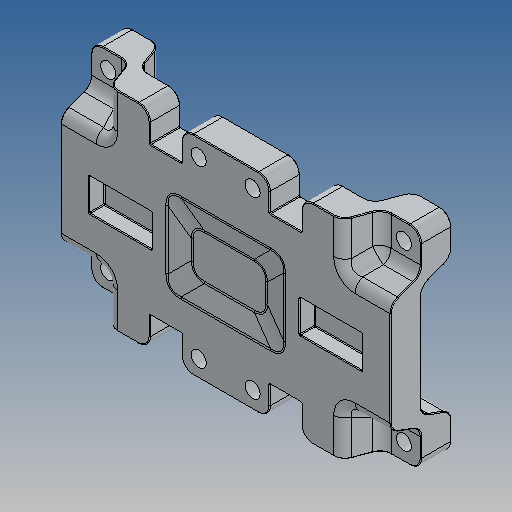
# Autodesk Inventor part: 84428-LtBluishGray
Saved by Autodesk Inventor 2025 (Build 290162010, 162A)
## iProperties
Created: 2024-11-28
Part Number: 84428-LtBluishGray
Material: ABS-Kunststoff
Document SubType Name: Modeling
Designer: hp.muther
Density: 1.06 g/cm^3
Appearance: LtBluishGray
Author: hp.muther
Autodesk Inventor part; units mm, degrees
(part 1 of 2)
ref_plane "YZ Plane" through (0, 0, 0) normal (1, 0, 0) x (0, 1, 0)
ref_plane "XZ Plane" through (0, 0, 0) normal (0, 1, 0) x (-1, 0, 0)
ref_plane "XY Plane" through (0, 0, 0) normal (0, 0, 1) x (1, 0, 0)
sketch "Skizze1" plane through (0, 0, 0) normal (0, 1, 0) x (-1, 0, 0)
  line L0 (0, 0) -> (0, 27.5)
  line L1 (0, 27.5) -> (43.5, 27.5)
  line L2 (43.5, 27.5) -> (43.5, 0)
  line L3 (43.5, 0) -> (0, 0)
  dimension "d0" = 27.5
  dimension "d1" = 43.5
  constraints: 8 end point, 3 perpendicular, 1 vertical
  measures "d0" distance of L0.start L0.end
  measures "d1" distance of L2.end L0.start
extrude "Extrusion1" add sketch "Skizze1" along normal blind 8
sketch "Skizze2" plane through (0, 8, 0) normal (0, 1, 0) x (1, 0, 0)
  line L0 (-43.5, 0) -> (-43.5, -27.5) projected
  line L1 (-43.5, -27.5) -> (0, -27.5) projected
  line L2 (-43.5, -27.5) -> (-30.5882, -27.5)
  line L3 (-30.5882, -27.5) -> (-30.5882, -14.5882)
  line L4 (-30.5882, -14.5882) -> (-43.5, -14.5882)
  line L5 (-43.5, -14.5882) -> (-43.5, -27.5)
  line L6 (-30.5882, -19.5) -> (-33.5, -27.5) construction
  point P0 (-43.5, -14.5882)
  dimension "d4" = 12.9118
  dimension "d10" = 20
  dimension "d11" = 8
  dimension "d12" = 10
  constraints: 10 end point, 2 parallel, 2 perpendicular, 2 point on line, 1 horizontal
  measures "d4" distance of L3.end L4.end
  measures "d10" angle of L3 L6
  measures "d11" vertical distance of L6.start L6.end
  measures "d12" distance from line of L6.end L0
extrude "Extrusion2" add sketch "Skizze2" along normal blind 8
draft "Flächenverjüngung1" angle 20 pull direction (0, 1, 0) faces at (-34.8922, 10.6667, 14.5882) (-30.5882, 10.6667, 23.1961) fixed edges at (-37.0441, 8, 14.5882) (-30.5882, 8, 21.0441)
sketch "Skizze3" plane through (0, 8, 0) normal (0, 1, 0) x (1, 0, 0)
  line L0 (-43.5, -27.5) -> (-33.5, -27.5)
  line L1 (-33.5, -27.5) -> (-33.5, -17.5)
  line L2 (-33.5, -17.5) -> (-43.5, -17.5)
  line L3 (-43.5, -17.5) -> (-43.5, -27.5)
  dimension "d13" = 10
  constraints: 8 end point, 2 parallel, 2 perpendicular, 1 horizontal
  measures "d13" distance of L1.end L2.end
extrude "Extrusion3" cut sketch "Skizze3" against normal blind 8 draft 20
sketch "Skizze4" plane through (0, 0, 0) normal (0, -1, 0) x (1, 0, 0)
  line L0 (0, 0) -> (-43.5, 0) projected
  line L1 (0, 27.5) -> (0, 0) projected
  line L2 (-30.5882, 27.5) -> (0, 27.5) projected
  line L3 (-11.6, 27.5) -> (-20, 27.5)
  line L4 (-20, 27.5) -> (-20, 19.5)
  line L5 (-20, 19.5) -> (-11.6, 19.5)
  line L6 (-11.6, 19.5) -> (-11.6, 27.5)
  dimension "d16" = 19.5
  dimension "d17" = 8.4
  dimension "d18" = 20
  constraints: 8 end point, 2 parallel, 1 horizontal, 1 perpendicular, 1 point on line
  measures "d16" distance between parallel lines of L5 L0
  measures "d17" distance between parallel lines of L6 L4
  measures "d18" distance between parallel lines of L4 L1
extrude "Extrusion4" cut sketch "Skizze4" against normal through all
sketch "Skizze5" plane through (0, 0, 0) normal (0, -1, 0) x (1, 0, 0)
  line L0 (0, 0) -> (-43.5, 0) projected
  line L1 (0, 27.5) -> (0, 0) projected
  line L2 (-36, 0) -> (-19.5, 0)
  line L3 (-19.5, 0) -> (-19.5, 4.25)
  line L4 (-19.5, 4.25) -> (-36, 4.25)
  line L5 (-36, 4.25) -> (-36, 0)
  circle A0 centre (-7.1, 23) radius 2
  line L6 (-11.6, 27.5) -> (0, 27.5) projected
  line L7 (-11.6, 27.5) -> (-11.6, 19.5) projected
  dimension "d21" = 16.5
  dimension "d22" = 4.25
  dimension "d23" = 36
  dimension "d26" = 4
  dimension "d46" = 4.5
  dimension "d47" = 4.5
  constraints: 8 end point, 2 parallel, 1 centre point, 1 horizontal, 1 perpendicular, 1 point on line
  measures "d21" distance of L3.end L4.end
  measures "d22" distance between parallel lines of L0 L4
  measures "d23" distance between parallel lines of L5 L1
  measures "d26" diameter of A0
  measures "d46" distance from line of A0.centre L6
  measures "d47" distance from line of A0.centre L7
extrude "Extrusion5" cut sketch "Skizze5" against normal blind 4
sketch "Skizze6" plane through (0, 0, 0) normal (0, -1, 0) x (1, 0, 0)
  line L0 (0, 0) -> (-19.5, 0) projected
  line L1 (0, 27.5) -> (0, 0) projected
  line L2 (0, 0) -> (-9.8287, 0)
  line L3 (-9.8287, 0) -> (-9.8287, 5.8287)
  line L4 (-9.8287, 5.8287) -> (0, 5.8287)
  line L5 (0, 5.8287) -> (0, 0)
  line L6 (0, 0) -> (-15.5, 0)
  line L7 (-15.5, 0) -> (-15.5, 11.5)
  line L8 (-15.5, 11.5) -> (0, 11.5)
  line L9 (0, 11.5) -> (0, 0)
  line L10 (-15.5, 0) -> (-9.8287, 1)
  point P0 (0, 5.8287)
  point P1 (-9.8287, 0)
  dimension "d29" = 9.8287
  dimension "d30" = 5.8287
  dimension "d34" = 11.5
  dimension "d35" = 15.5
  dimension "d36" = 10
  dimension "d37" = 1
  dimension "d38" = 7.5475
  dimension "d39" = 5.6713
  constraints: 18 end point, 4 parallel, 2 horizontal, 2 perpendicular, 1 point on line
  measures "d29" distance of L3.end L4.end
  measures "d30" distance of L2.end L3.end
  measures "d34" distance between parallel lines of L0 L8
  measures "d35" distance between parallel lines of L9 L7
  measures "d36" angle of L6 L10
  measures "d37" distance from line of L0 L10.end
  measures "d39" distance between parallel lines of L8 L4
extrude "Extrusion6" cut sketch "Skizze6" against normal blind 1 contours L0 L3 L4 L1
draft "Flächenverjüngung2" angle 80 pull direction (0, -1, 0) faces at (-9.8287, 0.3333, 3.8858) (-3.2762, 0.6667, 5.8287) fixed edges at (-9.8287, 1, 2.9144) (-4.9144, 1, 5.8287)
fillet "Rundung1" radius 20 1 edges at (-12.6644, 0.5, 8.6644)
mirror "Spiegeln1" about plane through (-7.1, 4, 23) normal (0, -1, 0) of "Extrusion6", "Flächenverjüngung2", "Rundung1"
sketch "Skizze7" plane through (0, 8, 0) normal (0, -1, 0) x (1, 0, 0)
  line L0 (-43.5, 27.5) -> (-33.5, 27.5) projected
  line L1 (-43.5, 17.5) -> (-43.5, 27.5) projected
  circle A0 centre (-39, 23) radius 2
  point P0 (0, 0)
  dimension "d41" = 4
  dimension "d42" = 4.5
  dimension "d43" = 4.5
  constraints: 1 centre point
  measures "d41" diameter of A0
  measures "d42" distance from line of A0.centre L1
  measures "d43" distance from line of A0.centre L0
extrude "Extrusion7" cut sketch "Skizze7" against normal blind 4
fillet "Rundung2" radius 3 25 edges at (-30.5882, 8, 21.0441) (-37.0441, 8, 14.5882) (-32.0441, 12, 16.0441) (-38.5, 16, 17.5) (-33.5, 16, 22.5) (-38.5, 8, 17.5) (-33.5, 8, 22.5) (-32.0441, 4, 16.0441) (-30.5882, 0, 21.0441) (-37.0441, 0, 14.5882) (-43.5, 12, 27.5) (-20, 4, 27.5) (-11.6, 4, 27.5) (-14.6285, 8, 10.6285) (-15.5, 8, 4.0135) (-6.0135, 8, 11.5) (-3.1779, 7, 5.8287) (-9.8287, 7, 1.1779) (-8.9572, 7, 4.9572) (-15.5, 0, 4.0135) (-6.0135, 0, 11.5) (-14.6285, 0, 10.6285) (-9.8287, 1, 1.1779) (-3.1779, 1, 5.8287) (-8.9572, 1, 4.9572)
fillet "Rundung2" radius 0.2 4 edges at (-20, 4, 19.5) (-11.6, 4, 19.5) (-19.5, 2, 4.25) (-36, 2, 4.25)
fillet "Rundung3" radius 0.2 48 edges at (-20.8787, 8, 26.6213) (-20, 8, 22.1) (-19.9414, 8, 19.5586) (-15.8, 8, 19.5) (-11.6586, 8, 19.5586) (-11.6, 8, 22.1) (-10.7213, 8, 26.6213) (-4.3, 8, 27.5) (-30.2083, 8.5425, 27.5) (-32.0441, 12, 27.5) (-33.8799, 15.4575, 27.5) (-38.0503, 16, 27.5) (-42.6213, 16, 26.6213) (-43.5, 16, 22.0503) (-43.5, 15.4575, 17.8799) (-43.5, 12, 16.0441) (-43.5, 8.5425, 14.2083) (-43.5, 8, 6.2438) (-25.7438, 8, 27.5) (-20.8787, 0, 26.6213) (-20, 0, 22.1) (-19.9414, 0, 19.5586) (-15.8, 0, 19.5) (-11.6586, 0, 19.5586) (-11.6, 0, 22.1) (-10.7213, 0, 26.6213) (-4.3, 0, 27.5) (-30.2083, 0.5425, 27.5) (-32.0441, 4, 27.5) (-33.8799, 7.4575, 27.5) (-38.0503, 8, 27.5) (-42.6213, 8, 26.6213) (-43.5, 8, 22.0503) (-43.5, 7.4575, 17.8799) (-43.5, 4, 16.0441) (-43.5, 0.5425, 14.2083) (-43.5, 0, 6.2438) (-25.7438, 0, 27.5) (-19.5586, 0, 4.1914) (-19.5, 0, 2.025) (-35.9414, 0, 4.1914) (-36, 0, 2.025) (-27.75, 0, 4.25) (-19.5586, 4, 4.1914) (-19.5, 4, 2.025) (-35.9414, 4, 4.1914) (-36, 4, 2.025) (-27.75, 4, 4.25)
mirror "Spiegeln2" about plane through (0, 0, 0) normal (0, 0, -1)
mirror "Spiegeln3" about plane through (0, 0, 27.5) normal (1, 0, 0)
sketch "Skizze8" plane through (0, 8, 0) normal (0, 1, 0) x (1, 0, 0)
  line L0 (-32, -5) -> (-42, -5)
  line L1 (-42, -5) -> (-42, 5)
  line L2 (-42, 5) -> (-32, 5)
  line L3 (-32, 5) -> (-32, -5)
  line L4 (-41.9167, -4.9167) -> (-41.9167, 4.9167)
  line L5 (-41.9167, 4.9167) -> (-32.0833, 4.9167)
  line L6 (-32.0833, 4.9167) -> (-32.0833, -4.9167)
  line L7 (-32.0833, -4.9167) -> (-41.9167, -4.9167)
  spline S0 degree 3 poles (-35.473, -0.7347) (-35.3624, -0.6395) (-35.2195, -0.4588) (-35.1278, -0.1698) (-35.0916, 0.0842) (-35.1043, 0.3702) (-35.1747, 0.6728) (-35.3516, 1.0506) (-35.5547, 1.2912) (-35.7186, 1.4187) knots 0 0 0 0 0.178983 0.273938 0.368222 0.492079 0.622193 0.746013 1 1 1 1
  line L8 (-35.473, -0.7347) -> (-35.3624, -0.6395) construction
  line L9 (-35.3624, -0.6395) -> (-35.2195, -0.4588) construction
  line L10 (-35.2195, -0.4588) -> (-35.1278, -0.1698) construction
  line L11 (-35.1278, -0.1698) -> (-35.0916, 0.0842) construction
  line L12 (-35.0916, 0.0842) -> (-35.1043, 0.3702) construction
  line L13 (-35.1043, 0.3702) -> (-35.1747, 0.6728) construction
  line L14 (-35.1747, 0.6728) -> (-35.3516, 1.0506) construction
  line L15 (-35.3516, 1.0506) -> (-35.5547, 1.2912) construction
  line L16 (-35.5547, 1.2912) -> (-35.7186, 1.4187) construction
  spline S1 degree 3 poles (-35.3027, 1.3649) (-35.2254, 1.2746) (-35.09, 1.0821) (-34.9632, 0.8118) (-34.8957, 0.5786) (-34.8526, 0.3435) (-34.8424, 0.119) (-34.8636, -0.0901) (-34.8884, -0.224) (-34.9248, -0.3582) (-34.9903, -0.5271) (-35.0674, -0.6551) (-35.1272, -0.7328) (-35.137, -0.7452) knots 0 0 0 0 0.159789 0.316619 0.39902 0.481421 0.638299 0.698008 0.757718 0.817853 0.877988 0.980322 1 1 1 1
  line L17 (-35.3027, 1.3649) -> (-35.2254, 1.2746) construction
  line L18 (-35.2254, 1.2746) -> (-35.09, 1.0821) construction
  line L19 (-35.09, 1.0821) -> (-34.9632, 0.8118) construction
  line L20 (-34.9632, 0.8118) -> (-34.8957, 0.5786) construction
  line L21 (-34.8957, 0.5786) -> (-34.8526, 0.3435) construction
  line L22 (-34.8526, 0.3435) -> (-34.8424, 0.119) construction
  line L23 (-34.8424, 0.119) -> (-34.8636, -0.0901) construction
  line L24 (-34.8636, -0.0901) -> (-34.8884, -0.224) construction
  line L25 (-34.8884, -0.224) -> (-34.9248, -0.3582) construction
  line L26 (-34.9248, -0.3582) -> (-34.9903, -0.5271) construction
  line L27 (-34.9903, -0.5271) -> (-35.0674, -0.6551) construction
  line L28 (-35.0674, -0.6551) -> (-35.1272, -0.7328) construction
  line L29 (-35.1272, -0.7328) -> (-35.137, -0.7452) construction
  spline S2 degree 3 poles (-38.4765, 2.1644) (-38.496, 2.156) (-38.5452, 2.1307) (-38.6253, 2.0736) (-38.7157, 1.9854) (-38.8087, 1.8699) (-38.8816, 1.7254) (-38.9348, 1.5546) (-38.9716, 1.3719) (-38.9833, 1.1731) (-38.9859, 0.9738) (-38.959, 0.783) (-38.9219, 0.6128) (-38.8748, 0.4674) (-38.8227, 0.3417) (-38.748, 0.2091) (-38.682, 0.1256) (-38.6415, 0.0726) knots 0 0 0 0 0.027057 0.070486 0.124946 0.187916 0.258874 0.330051 0.415845 0.496025 0.584026 0.669773 0.741314 0.806204 0.86459 0.914785 1 1 1 1
  line L30 (-38.4765, 2.1644) -> (-38.496, 2.156) construction
  line L31 (-38.496, 2.156) -> (-38.5452, 2.1307) construction
  line L32 (-38.5452, 2.1307) -> (-38.6253, 2.0736) construction
  line L33 (-38.6253, 2.0736) -> (-38.7157, 1.9854) construction
  line L34 (-38.7157, 1.9854) -> (-38.8087, 1.8699) construction
  line L35 (-38.8087, 1.8699) -> (-38.8816, 1.7254) construction
  line L36 (-38.8816, 1.7254) -> (-38.9348, 1.5546) construction
  line L37 (-38.9348, 1.5546) -> (-38.9716, 1.3719) construction
  line L38 (-38.9716, 1.3719) -> (-38.9833, 1.1731) construction
  line L39 (-38.9833, 1.1731) -> (-38.9859, 0.9738) construction
  line L40 (-38.9859, 0.9738) -> (-38.959, 0.783) construction
  line L41 (-38.959, 0.783) -> (-38.9219, 0.6128) construction
  line L42 (-38.9219, 0.6128) -> (-38.8748, 0.4674) construction
  line L43 (-38.8748, 0.4674) -> (-38.8227, 0.3417) construction
  line L44 (-38.8227, 0.3417) -> (-38.748, 0.2091) construction
  line L45 (-38.748, 0.2091) -> (-38.682, 0.1256) construction
  line L46 (-38.682, 0.1256) -> (-38.6415, 0.0726) construction
  spline S3 degree 3 poles (-38.973, 0.104) (-38.9979, 0.1432) (-39.0496, 0.2355) (-39.0988, 0.3548) (-39.1347, 0.4582) (-39.1607, 0.5455) (-39.1829, 0.6361) (-39.2024, 0.7334) (-39.2194, 0.8381) (-39.2317, 0.9573) (-39.2347, 1.0772) (-39.2319, 1.1851) (-39.227, 1.2895) (-39.2167, 1.4009) (-39.1978, 1.5159) (-39.1663, 1.6523) (-39.1252, 1.7852) (-39.0668, 1.9143) (-39.0137, 2.0064) (-38.9537, 2.0889) (-38.9024, 2.1484) (-38.8687, 2.1839) (-38.8557, 2.1969) knots 0 0 0 0 0.059837 0.132225 0.172452 0.212678 0.257027 0.301377 0.354532 0.407687 0.46224 0.516793 0.566497 0.616202 0.669387 0.722571 0.810819 0.854806 0.898794 0.93783 0.976866 1 1 1 1
  line L47 (-38.973, 0.104) -> (-38.9979, 0.1432) construction
  line L48 (-38.9979, 0.1432) -> (-39.0496, 0.2355) construction
  line L49 (-39.0496, 0.2355) -> (-39.0988, 0.3548) construction
  line L50 (-39.0988, 0.3548) -> (-39.1347, 0.4582) construction
  line L51 (-39.1347, 0.4582) -> (-39.1607, 0.5455) construction
  line L52 (-39.1607, 0.5455) -> (-39.1829, 0.6361) construction
  line L53 (-39.1829, 0.6361) -> (-39.2024, 0.7334) construction
  line L54 (-39.2024, 0.7334) -> (-39.2194, 0.8381) construction
  line L55 (-39.2194, 0.8381) -> (-39.2317, 0.9573) construction
  line L56 (-39.2317, 0.9573) -> (-39.2347, 1.0772) construction
  line L57 (-39.2347, 1.0772) -> (-39.2319, 1.1851) construction
  line L58 (-39.2319, 1.1851) -> (-39.227, 1.2895) construction
  line L59 (-39.227, 1.2895) -> (-39.2167, 1.4009) construction
  line L60 (-39.2167, 1.4009) -> (-39.1978, 1.5159) construction
  line L61 (-39.1978, 1.5159) -> (-39.1663, 1.6523) construction
  line L62 (-39.1663, 1.6523) -> (-39.1252, 1.7852) construction
  line L63 (-39.1252, 1.7852) -> (-39.0668, 1.9143) construction
  line L64 (-39.0668, 1.9143) -> (-39.0137, 2.0064) construction
  line L65 (-39.0137, 2.0064) -> (-38.9537, 2.0889) construction
  line L66 (-38.9537, 2.0889) -> (-38.9024, 2.1484) construction
  line L67 (-38.9024, 2.1484) -> (-38.8687, 2.1839) construction
  line L68 (-38.8687, 2.1839) -> (-38.8557, 2.1969) construction
  spline S4 degree 3 poles (-36.653, 0.7792) (-36.6576, 0.6963) (-36.7122, 0.5242) (-36.8901, 0.5099) (-36.9901, 0.5385) (-37.0893, 0.5769) (-37.1802, 0.6371) (-37.2609, 0.726) (-37.3082, 0.8385) (-37.3294, 0.9568) (-37.3399, 1.0766) (-37.339, 1.2043) (-37.3177, 1.3389) (-37.2557, 1.4577) (-37.1613, 1.5412) (-37.0413, 1.5828) (-36.9075, 1.5817) (-36.7579, 1.5657) (-36.5824, 1.5258) (-36.391, 1.4628) (-36.1893, 1.374) (-35.9783, 1.2471) (-35.7808, 1.0856) (-35.6257, 0.8856) (-35.5009, 0.6796) (-35.43, 0.4656) (-35.4032, 0.2478) (-35.3962, 0.0501) (-35.4357, -0.1532) (-35.5185, -0.3428) (-35.6607, -0.5088) (-35.8941, -0.634) (-36.1782, -0.6714) (-36.4895, -0.6312) (-36.7559, -0.5759) (-37.0415, -0.4903) (-37.2985, -0.3989) (-37.5745, -0.2896) (-37.8049, -0.1786) (-38.0112, -0.0619) (-38.1801, 0.0538) (-38.3524, 0.1963) (-38.4952, 0.3757) (-38.6003, 0.5957) (-38.656, 0.8014) (-38.6787, 1.0207) (-38.672, 1.2395) (-38.6426, 1.471) (-38.5689, 1.6832) (-38.4342, 1.8427) (-38.2496, 1.9328) (-38.0438, 1.9273) (-37.8337, 1.893) (-37.655, 1.7906) (-37.5297, 1.6397) (-37.4854, 1.4696) (-37.4764, 1.317) (-37.5071, 1.1986) (-37.5522, 1.1238) (-37.6077, 1.0813) (-37.6746, 1.0656) (-37.7498, 1.0726) (-37.8285, 1.0877) (-37.8988, 1.1301) (-37.9872, 1.1175) (-38.024, 1.0355) (-38.0262, 0.9522) (-38.0081, 0.8654) (-37.9569, 0.7893) (-37.8896, 0.7032) (-37.7734, 0.6342) (-37.6311, 0.5633) (-37.4707, 0.4893) (-37.2636, 0.4036) (-37.021, 0.3163) (-36.746, 0.2176) (-36.5084, 0.1557) (-36.3238, 0.1341) (-36.193, 0.1683) (-36.1433, 0.28) (-36.1489, 0.4008) (-36.2089, 0.5256) (-36.3468, 0.6608) (-36.4774, 0.7295) (-36.5685, 0.7576) knots 0 0 0 0 0.019628 0.027018 0.033965 0.040941 0.048656 0.056022 0.065138 0.073134 0.080528 0.089672 0.099198 0.108096 0.11648 0.124306 0.133455 0.143566 0.155056 0.170131 0.184678 0.199975 0.220335 0.236354 0.251449 0.269379 0.28185 0.296238 0.309598 0.323802 0.338076 0.353381 0.376853 0.395227 0.417369 0.432365 0.456106 0.473078 0.492988 0.508303 0.521448 0.534776 0.553874 0.56769 0.58436 0.597126 0.612617 0.628953 0.644733 0.657749 0.670618 0.685183 0.698991 0.713855 0.726199 0.737953 0.749129 0.757115 0.762561 0.766674 0.771046 0.776214 0.782044 0.787215 0.792824 0.7976 0.804046 0.809875 0.815303 0.822628 0.832017 0.842463 0.855224 0.868048 0.888264 0.907855 0.927805 0.938062 0.946095 0.95306 0.961017 0.970332 0.980566 1 1 1 1
  line L69 (-36.653, 0.7792) -> (-36.6576, 0.6963) construction
  line L70 (-36.6576, 0.6963) -> (-36.7122, 0.5242) construction
  line L71 (-36.7122, 0.5242) -> (-36.8901, 0.5099) construction
  line L72 (-36.8901, 0.5099) -> (-36.9901, 0.5385) construction
  line L73 (-36.9901, 0.5385) -> (-37.0893, 0.5769) construction
  line L74 (-37.0893, 0.5769) -> (-37.1802, 0.6371) construction
  line L75 (-37.1802, 0.6371) -> (-37.2609, 0.726) construction
  line L76 (-37.2609, 0.726) -> (-37.3082, 0.8385) construction
  line L77 (-37.3082, 0.8385) -> (-37.3294, 0.9568) construction
  line L78 (-37.3294, 0.9568) -> (-37.3399, 1.0766) construction
  line L79 (-37.3399, 1.0766) -> (-37.339, 1.2043) construction
  line L80 (-37.339, 1.2043) -> (-37.3177, 1.3389) construction
  line L81 (-37.3177, 1.3389) -> (-37.2557, 1.4577) construction
  line L82 (-37.2557, 1.4577) -> (-37.1613, 1.5412) construction
  line L83 (-37.1613, 1.5412) -> (-37.0413, 1.5828) construction
  line L84 (-37.0413, 1.5828) -> (-36.9075, 1.5817) construction
  line L85 (-36.9075, 1.5817) -> (-36.7579, 1.5657) construction
  line L86 (-36.7579, 1.5657) -> (-36.5824, 1.5258) construction
  line L87 (-36.5824, 1.5258) -> (-36.391, 1.4628) construction
  line L88 (-36.391, 1.4628) -> (-36.1893, 1.374) construction
  line L89 (-36.1893, 1.374) -> (-35.9783, 1.2471) construction
  line L90 (-35.9783, 1.2471) -> (-35.7808, 1.0856) construction
  line L91 (-35.7808, 1.0856) -> (-35.6257, 0.8856) construction
  line L92 (-35.6257, 0.8856) -> (-35.5009, 0.6796) construction
  line L93 (-35.5009, 0.6796) -> (-35.43, 0.4656) construction
  line L94 (-35.43, 0.4656) -> (-35.4032, 0.2478) construction
  line L95 (-35.4032, 0.2478) -> (-35.3962, 0.0501) construction
  line L96 (-35.3962, 0.0501) -> (-35.4357, -0.1532) construction
  line L97 (-35.4357, -0.1532) -> (-35.5185, -0.3428) construction
  line L98 (-35.5185, -0.3428) -> (-35.6607, -0.5088) construction
  line L99 (-35.6607, -0.5088) -> (-35.8941, -0.634) construction
  line L100 (-35.8941, -0.634) -> (-36.1782, -0.6714) construction
  line L101 (-36.1782, -0.6714) -> (-36.4895, -0.6312) construction
  line L102 (-36.4895, -0.6312) -> (-36.7559, -0.5759) construction
  line L103 (-36.7559, -0.5759) -> (-37.0415, -0.4903) construction
  line L104 (-37.0415, -0.4903) -> (-37.2985, -0.3989) construction
  line L105 (-37.2985, -0.3989) -> (-37.5745, -0.2896) construction
  line L106 (-37.5745, -0.2896) -> (-37.8049, -0.1786) construction
  line L107 (-37.8049, -0.1786) -> (-38.0112, -0.0619) construction
  line L108 (-38.0112, -0.0619) -> (-38.1801, 0.0538) construction
  line L109 (-38.1801, 0.0538) -> (-38.3524, 0.1963) construction
  line L110 (-38.3524, 0.1963) -> (-38.4952, 0.3757) construction
  line L111 (-38.4952, 0.3757) -> (-38.6003, 0.5957) construction
  line L112 (-38.6003, 0.5957) -> (-38.656, 0.8014) construction
  line L113 (-38.656, 0.8014) -> (-38.6787, 1.0207) construction
  line L114 (-38.6787, 1.0207) -> (-38.672, 1.2395) construction
  line L115 (-38.672, 1.2395) -> (-38.6426, 1.471) construction
  line L116 (-38.6426, 1.471) -> (-38.5689, 1.6832) construction
  line L117 (-38.5689, 1.6832) -> (-38.4342, 1.8427) construction
  line L118 (-38.4342, 1.8427) -> (-38.2496, 1.9328) construction
  line L119 (-38.2496, 1.9328) -> (-38.0438, 1.9273) construction
  line L120 (-38.0438, 1.9273) -> (-37.8337, 1.893) construction
  line L121 (-37.8337, 1.893) -> (-37.655, 1.7906) construction
  line L122 (-37.655, 1.7906) -> (-37.5297, 1.6397) construction
  line L123 (-37.5297, 1.6397) -> (-37.4854, 1.4696) construction
  line L124 (-37.4854, 1.4696) -> (-37.4764, 1.317) construction
  line L125 (-37.4764, 1.317) -> (-37.5071, 1.1986) construction
  line L126 (-37.5071, 1.1986) -> (-37.5522, 1.1238) construction
  line L127 (-37.5522, 1.1238) -> (-37.6077, 1.0813) construction
  line L128 (-37.6077, 1.0813) -> (-37.6746, 1.0656) construction
  line L129 (-37.6746, 1.0656) -> (-37.7498, 1.0726) construction
  line L130 (-37.7498, 1.0726) -> (-37.8285, 1.0877) construction
  line L131 (-37.8285, 1.0877) -> (-37.8988, 1.1301) construction
  line L132 (-37.8988, 1.1301) -> (-37.9872, 1.1175) construction
  line L133 (-37.9872, 1.1175) -> (-38.024, 1.0355) construction
  line L134 (-38.024, 1.0355) -> (-38.0262, 0.9522) construction
  line L135 (-38.0262, 0.9522) -> (-38.0081, 0.8654) construction
  line L136 (-38.0081, 0.8654) -> (-37.9569, 0.7893) construction
  line L137 (-37.9569, 0.7893) -> (-37.8896, 0.7032) construction
  line L138 (-37.8896, 0.7032) -> (-37.7734, 0.6342) construction
  line L139 (-37.7734, 0.6342) -> (-37.6311, 0.5633) construction
  line L140 (-37.6311, 0.5633) -> (-37.4707, 0.4893) construction
  line L141 (-37.4707, 0.4893) -> (-37.2636, 0.4036) construction
  line L142 (-37.2636, 0.4036) -> (-37.021, 0.3163) construction
  line L143 (-37.021, 0.3163) -> (-36.746, 0.2176) construction
  line L144 (-36.746, 0.2176) -> (-36.5084, 0.1557) construction
  line L145 (-36.5084, 0.1557) -> (-36.3238, 0.1341) construction
  line L146 (-36.3238, 0.1341) -> (-36.193, 0.1683) construction
  line L147 (-36.193, 0.1683) -> (-36.1433, 0.28) construction
  line L148 (-36.1433, 0.28) -> (-36.1489, 0.4008) construction
  line L149 (-36.1489, 0.4008) -> (-36.2089, 0.5256) construction
  line L150 (-36.2089, 0.5256) -> (-36.3468, 0.6608) construction
  line L151 (-36.3468, 0.6608) -> (-36.4774, 0.7295) construction
  line L152 (-36.4774, 0.7295) -> (-36.5685, 0.7576) construction
  spline S5 degree 3 poles (-36.5685, 0.7576) (-36.4774, 0.7295) (-36.3468, 0.6608) (-36.2089, 0.5256) (-36.1489, 0.4008) (-36.1433, 0.28) (-36.193, 0.1683) (-36.3238, 0.1341) (-36.5084, 0.1557) (-36.746, 0.2176) (-37.021, 0.3163) (-37.2636, 0.4036) (-37.4707, 0.4893) (-37.6311, 0.5633) (-37.7734, 0.6342) (-37.8896, 0.7032) (-37.9569, 0.7893) (-38.0081, 0.8654) (-38.0262, 0.9522) (-38.024, 1.0355) (-37.9872, 1.1175) (-37.8988, 1.1301) (-37.8285, 1.0877) (-37.7498, 1.0726) (-37.6746, 1.0656) (-37.6077, 1.0813) (-37.5522, 1.1238) (-37.5071, 1.1986) (-37.4764, 1.317) (-37.4854, 1.4696) (-37.5297, 1.6397) (-37.655, 1.7906) (-37.8337, 1.893) (-38.0438, 1.9273) (-38.2496, 1.9328) (-38.4342, 1.8427) (-38.5689, 1.6832) (-38.6426, 1.471) (-38.672, 1.2395) (-38.6787, 1.0207) (-38.656, 0.8014) (-38.6003, 0.5957) (-38.4952, 0.3757) (-38.3524, 0.1963) (-38.1801, 0.0538) (-38.0112, -0.0619) (-37.8049, -0.1786) (-37.5745, -0.2896) (-37.2985, -0.3989) (-37.0415, -0.4903) (-36.7559, -0.5759) (-36.4895, -0.6312) (-36.1782, -0.6714) (-35.8941, -0.634) (-35.6607, -0.5088) (-35.5185, -0.3428) (-35.4357, -0.1532) (-35.3962, 0.0501) (-35.4032, 0.2478) (-35.43, 0.4656) (-35.5009, 0.6796) (-35.6257, 0.8856) (-35.7808, 1.0856) (-35.9783, 1.2471) (-36.1893, 1.374) (-36.391, 1.4628) (-36.5824, 1.5258) (-36.7579, 1.5657) (-36.9075, 1.5817) (-37.0413, 1.5828) (-37.1613, 1.5412) (-37.2557, 1.4577) (-37.3177, 1.3389) (-37.339, 1.2043) (-37.3399, 1.0766) (-37.3294, 0.9568) (-37.3082, 0.8385) (-37.2609, 0.726) (-37.1802, 0.6371) (-37.0893, 0.5769) (-36.9901, 0.5385) (-36.8901, 0.5099) (-36.7122, 0.5242) (-36.6576, 0.6963) (-36.653, 0.7792) knots 0 0 0 0 0.019434 0.029668 0.038983 0.04694 0.053905 0.061938 0.072195 0.092145 0.111736 0.131952 0.144776 0.157537 0.167983 0.177372 0.184697 0.190125 0.195954 0.2024 0.207176 0.212785 0.217956 0.223786 0.228954 0.233326 0.237439 0.242885 0.250871 0.262047 0.273801 0.286145 0.301009 0.314817 0.329382 0.342251 0.355267 0.371047 0.387383 0.402874 0.41564 0.43231 0.446126 0.465224 0.478552 0.491697 0.507012 0.526922 0.543894 0.567635 0.582631 0.604773 0.623147 0.646619 0.661924 0.676198 0.690402 0.703762 0.71815 0.730621 0.748551 0.763646 0.779665 0.800025 0.815322 0.829869 0.844944 0.856434 0.866545 0.875694 0.88352 0.891904 0.900802 0.910328 0.919472 0.926866 0.934862 0.943978 0.951344 0.959059 0.966035 0.972982 0.980372 1 1 1 1
  line L153 (-36.5685, 0.7576) -> (-36.4774, 0.7295) construction
  line L154 (-36.4774, 0.7295) -> (-36.3468, 0.6608) construction
  line L155 (-36.3468, 0.6608) -> (-36.2089, 0.5256) construction
  line L156 (-36.2089, 0.5256) -> (-36.1489, 0.4008) construction
  line L157 (-36.1489, 0.4008) -> (-36.1433, 0.28) construction
  line L158 (-36.1433, 0.28) -> (-36.193, 0.1683) construction
  line L159 (-36.193, 0.1683) -> (-36.3238, 0.1341) construction
  line L160 (-36.3238, 0.1341) -> (-36.5084, 0.1557) construction
  line L161 (-36.5084, 0.1557) -> (-36.746, 0.2176) construction
  line L162 (-36.746, 0.2176) -> (-37.021, 0.3163) construction
  line L163 (-37.021, 0.3163) -> (-37.2636, 0.4036) construction
  line L164 (-37.2636, 0.4036) -> (-37.4707, 0.4893) construction
  line L165 (-37.4707, 0.4893) -> (-37.6311, 0.5633) construction
  line L166 (-37.6311, 0.5633) -> (-37.7734, 0.6342) construction
  line L167 (-37.7734, 0.6342) -> (-37.8896, 0.7032) construction
  line L168 (-37.8896, 0.7032) -> (-37.9569, 0.7893) construction
  line L169 (-37.9569, 0.7893) -> (-38.0081, 0.8654) construction
  line L170 (-38.0081, 0.8654) -> (-38.0262, 0.9522) construction
  line L171 (-38.0262, 0.9522) -> (-38.024, 1.0355) construction
  line L172 (-38.024, 1.0355) -> (-37.9872, 1.1175) construction
  line L173 (-37.9872, 1.1175) -> (-37.8988, 1.1301) construction
  line L174 (-37.8988, 1.1301) -> (-37.8285, 1.0877) construction
  line L175 (-37.8285, 1.0877) -> (-37.7498, 1.0726) construction
  line L176 (-37.7498, 1.0726) -> (-37.6746, 1.0656) construction
  line L177 (-37.6746, 1.0656) -> (-37.6077, 1.0813) construction
  line L178 (-37.6077, 1.0813) -> (-37.5522, 1.1238) construction
  line L179 (-37.5522, 1.1238) -> (-37.5071, 1.1986) construction
  line L180 (-37.5071, 1.1986) -> (-37.4764, 1.317) construction
  line L181 (-37.4764, 1.317) -> (-37.4854, 1.4696) construction
  line L182 (-37.4854, 1.4696) -> (-37.5297, 1.6397) construction
  line L183 (-37.5297, 1.6397) -> (-37.655, 1.7906) construction
  line L184 (-37.655, 1.7906) -> (-37.8337, 1.893) construction
  line L185 (-37.8337, 1.893) -> (-38.0438, 1.9273) construction
  line L186 (-38.0438, 1.9273) -> (-38.2496, 1.9328) construction
  line L187 (-38.2496, 1.9328) -> (-38.4342, 1.8427) construction
  line L188 (-38.4342, 1.8427) -> (-38.5689, 1.6832) construction
  line L189 (-38.5689, 1.6832) -> (-38.6426, 1.471) construction
  line L190 (-38.6426, 1.471) -> (-38.672, 1.2395) construction
  line L191 (-38.672, 1.2395) -> (-38.6787, 1.0207) construction
  line L192 (-38.6787, 1.0207) -> (-38.656, 0.8014) construction
  line L193 (-38.656, 0.8014) -> (-38.6003, 0.5957) construction
  line L194 (-38.6003, 0.5957) -> (-38.4952, 0.3757) construction
  line L195 (-38.4952, 0.3757) -> (-38.3524, 0.1963) construction
  line L196 (-38.3524, 0.1963) -> (-38.1801, 0.0538) construction
  line L197 (-38.1801, 0.0538) -> (-38.0112, -0.0619) construction
  line L198 (-38.0112, -0.0619) -> (-37.8049, -0.1786) construction
  line L199 (-37.8049, -0.1786) -> (-37.5745, -0.2896) construction
  line L200 (-37.5745, -0.2896) -> (-37.2985, -0.3989) construction
  line L201 (-37.2985, -0.3989) -> (-37.0415, -0.4903) construction
  line L202 (-37.0415, -0.4903) -> (-36.7559, -0.5759) construction
  line L203 (-36.7559, -0.5759) -> (-36.4895, -0.6312) construction
  line L204 (-36.4895, -0.6312) -> (-36.1782, -0.6714) construction
  line L205 (-36.1782, -0.6714) -> (-35.8941, -0.634) construction
  line L206 (-35.8941, -0.634) -> (-35.6607, -0.5088) construction
  line L207 (-35.6607, -0.5088) -> (-35.5185, -0.3428) construction
  line L208 (-35.5185, -0.3428) -> (-35.4357, -0.1532) construction
  line L209 (-35.4357, -0.1532) -> (-35.3962, 0.0501) construction
  line L210 (-35.3962, 0.0501) -> (-35.4032, 0.2478) construction
  line L211 (-35.4032, 0.2478) -> (-35.43, 0.4656) construction
  line L212 (-35.43, 0.4656) -> (-35.5009, 0.6796) construction
  line L213 (-35.5009, 0.6796) -> (-35.6257, 0.8856) construction
  line L214 (-35.6257, 0.8856) -> (-35.7808, 1.0856) construction
  line L215 (-35.7808, 1.0856) -> (-35.9783, 1.2471) construction
  line L216 (-35.9783, 1.2471) -> (-36.1893, 1.374) construction
  line L217 (-36.1893, 1.374) -> (-36.391, 1.4628) construction
  line L218 (-36.391, 1.4628) -> (-36.5824, 1.5258) construction
  line L219 (-36.5824, 1.5258) -> (-36.7579, 1.5657) construction
  line L220 (-36.7579, 1.5657) -> (-36.9075, 1.5817) construction
  line L221 (-36.9075, 1.5817) -> (-37.0413, 1.5828) construction
  line L222 (-37.0413, 1.5828) -> (-37.1613, 1.5412) construction
  line L223 (-37.1613, 1.5412) -> (-37.2557, 1.4577) construction
  line L224 (-37.2557, 1.4577) -> (-37.3177, 1.3389) construction
  line L225 (-37.3177, 1.3389) -> (-37.339, 1.2043) construction
  line L226 (-37.339, 1.2043) -> (-37.3399, 1.0766) construction
  line L227 (-37.3399, 1.0766) -> (-37.3294, 0.9568) construction
  line L228 (-37.3294, 0.9568) -> (-37.3082, 0.8385) construction
  line L229 (-37.3082, 0.8385) -> (-37.2609, 0.726) construction
  line L230 (-37.2609, 0.726) -> (-37.1802, 0.6371) construction
  line L231 (-37.1802, 0.6371) -> (-37.0893, 0.5769) construction
  line L232 (-37.0893, 0.5769) -> (-36.9901, 0.5385) construction
  line L233 (-36.9901, 0.5385) -> (-36.8901, 0.5099) construction
  line L234 (-36.8901, 0.5099) -> (-36.7122, 0.5242) construction
  line L235 (-36.7122, 0.5242) -> (-36.6576, 0.6963) construction
  line L236 (-36.6576, 0.6963) -> (-36.653, 0.7792) construction
  spline S6 degree 3 poles (-36.4459, 2.4614) (-36.659, 2.5126) (-37.0118, 2.6203) (-37.4792, 2.8097) (-37.7435, 2.9186) (-37.8615, 2.9876) knots 0 0 0 0 0.434487 0.729459 1 1 1 1
  line L237 (-36.4459, 2.4614) -> (-36.659, 2.5126) construction
  line L238 (-36.659, 2.5126) -> (-37.0118, 2.6203) construction
  line L239 (-37.0118, 2.6203) -> (-37.4792, 2.8097) construction
  line L240 (-37.4792, 2.8097) -> (-37.7435, 2.9186) construction
  line L241 (-37.7435, 2.9186) -> (-37.8615, 2.9876) construction
  spline S7 degree 3 poles (-37.8615, 2.9876) (-37.8896, 3.004) (-37.9483, 3.0417) (-38.008, 3.1224) (-38.013, 3.2088) (-38.0172, 3.2823) (-37.9686, 3.355) (-37.867, 3.3615) (-37.7329, 3.3463) (-37.555, 3.298) (-37.3426, 3.2417) (-37.1448, 3.173) (-36.9458, 3.1066) (-36.7442, 3.0312) (-36.534, 2.9393) (-36.3445, 2.8534) (-36.1878, 2.7622) (-36.1364, 2.6314) (-36.1459, 2.5251) (-36.2475, 2.422) (-36.3751, 2.4459) (-36.4459, 2.4614) knots 0 0 0 0 0.033985 0.073024 0.098291 0.123366 0.14909 0.179483 0.222309 0.292562 0.370552 0.452514 0.511152 0.58996 0.677574 0.750224 0.809779 0.859921 0.887962 0.916689 1 1 1 1
  line L242 (-37.8615, 2.9876) -> (-37.8896, 3.004) construction
  line L243 (-37.8896, 3.004) -> (-37.9483, 3.0417) construction
  line L244 (-37.9483, 3.0417) -> (-38.008, 3.1224) construction
  line L245 (-38.008, 3.1224) -> (-38.013, 3.2088) construction
  line L246 (-38.013, 3.2088) -> (-38.0172, 3.2823) construction
  line L247 (-38.0172, 3.2823) -> (-37.9686, 3.355) construction
  line L248 (-37.9686, 3.355) -> (-37.867, 3.3615) construction
  line L249 (-37.867, 3.3615) -> (-37.7329, 3.3463) construction
  line L250 (-37.7329, 3.3463) -> (-37.555, 3.298) construction
  line L251 (-37.555, 3.298) -> (-37.3426, 3.2417) construction
  line L252 (-37.3426, 3.2417) -> (-37.1448, 3.173) construction
  line L253 (-37.1448, 3.173) -> (-36.9458, 3.1066) construction
  line L254 (-36.9458, 3.1066) -> (-36.7442, 3.0312) construction
  line L255 (-36.7442, 3.0312) -> (-36.534, 2.9393) construction
  line L256 (-36.534, 2.9393) -> (-36.3445, 2.8534) construction
  line L257 (-36.3445, 2.8534) -> (-36.1878, 2.7622) construction
  line L258 (-36.1878, 2.7622) -> (-36.1364, 2.6314) construction
  line L259 (-36.1364, 2.6314) -> (-36.1459, 2.5251) construction
  line L260 (-36.1459, 2.5251) -> (-36.2475, 2.422) construction
  line L261 (-36.2475, 2.422) -> (-36.3751, 2.4459) construction
  line L262 (-36.3751, 2.4459) -> (-36.4459, 2.4614) construction
  spline S8 degree 3 poles (-37.3796, 4.0448) (-37.3842, 4.0458) (-37.5051, 4.0724) (-37.7312, 4.117) (-38.0573, 4.1207) (-38.3379, 4.0482) (-38.5493, 3.8654) (-38.6556, 3.6202) (-38.6743, 3.349) (-38.663, 3.0937) (-38.6019, 2.841) (-38.4734, 2.5938) (-38.2617, 2.3709) (-37.9712, 2.2001) (-37.6624, 2.0624) (-37.3426, 1.934) (-37.0239, 1.8314) (-36.8076, 1.7667) (-36.6984, 1.741) knots 0 0 0 0 0.00314 0.081594 0.151661 0.21734 0.267618 0.330698 0.387833 0.446036 0.498881 0.558118 0.627934 0.69858 0.779055 0.85117 0.925881 1 1 1 1
  line L263 (-37.3796, 4.0448) -> (-37.3842, 4.0458) construction
  line L264 (-37.3842, 4.0458) -> (-37.5051, 4.0724) construction
  line L265 (-37.5051, 4.0724) -> (-37.7312, 4.117) construction
  line L266 (-37.7312, 4.117) -> (-38.0573, 4.1207) construction
  line L267 (-38.0573, 4.1207) -> (-38.3379, 4.0482) construction
  line L268 (-38.3379, 4.0482) -> (-38.5493, 3.8654) construction
  line L269 (-38.5493, 3.8654) -> (-38.6556, 3.6202) construction
  line L270 (-38.6556, 3.6202) -> (-38.6743, 3.349) construction
  line L271 (-38.6743, 3.349) -> (-38.663, 3.0937) construction
  line L272 (-38.663, 3.0937) -> (-38.6019, 2.841) construction
  line L273 (-38.6019, 2.841) -> (-38.4734, 2.5938) construction
  line L274 (-38.4734, 2.5938) -> (-38.2617, 2.3709) construction
  line L275 (-38.2617, 2.3709) -> (-37.9712, 2.2001) construction
  line L276 (-37.9712, 2.2001) -> (-37.6624, 2.0624) construction
  line L277 (-37.6624, 2.0624) -> (-37.3426, 1.934) construction
  line L278 (-37.3426, 1.934) -> (-37.0239, 1.8314) construction
  line L279 (-37.0239, 1.8314) -> (-36.8076, 1.7667) construction
  line L280 (-36.8076, 1.7667) -> (-36.6984, 1.741) construction
  spline S9 degree 3 poles (-37.3796, 4.0448) (-37.3842, 4.0458) (-37.5051, 4.0724) (-37.7312, 4.117) (-38.0573, 4.1207) (-38.3379, 4.0482) (-38.5493, 3.8654) (-38.6556, 3.6202) (-38.6743, 3.349) (-38.663, 3.0937) (-38.6019, 2.841) (-38.4734, 2.5938) (-38.2617, 2.3709) (-37.9712, 2.2001) (-37.6624, 2.0624) (-37.3426, 1.934) (-37.0239, 1.8314) (-36.8076, 1.7667) (-36.6984, 1.741) knots 0 0 0 0 0.00314 0.081594 0.151661 0.21734 0.267618 0.330698 0.387833 0.446036 0.498881 0.558118 0.627934 0.69858 0.779055 0.85117 0.925881 1 1 1 1
  line L281 (-37.3796, 4.0448) -> (-37.3842, 4.0458) construction
  line L282 (-37.3842, 4.0458) -> (-37.5051, 4.0724) construction
  line L283 (-37.5051, 4.0724) -> (-37.7312, 4.117) construction
  line L284 (-37.7312, 4.117) -> (-38.0573, 4.1207) construction
  line L285 (-38.0573, 4.1207) -> (-38.3379, 4.0482) construction
  line L286 (-38.3379, 4.0482) -> (-38.5493, 3.8654) construction
  line L287 (-38.5493, 3.8654) -> (-38.6556, 3.6202) construction
  line L288 (-38.6556, 3.6202) -> (-38.6743, 3.349) construction
  line L289 (-38.6743, 3.349) -> (-38.663, 3.0937) construction
  line L290 (-38.663, 3.0937) -> (-38.6019, 2.841) construction
  line L291 (-38.6019, 2.841) -> (-38.4734, 2.5938) construction
  line L292 (-38.4734, 2.5938) -> (-38.2617, 2.3709) construction
  line L293 (-38.2617, 2.3709) -> (-37.9712, 2.2001) construction
  line L294 (-37.9712, 2.2001) -> (-37.6624, 2.0624) construction
  line L295 (-37.6624, 2.0624) -> (-37.3426, 1.934) construction
  line L296 (-37.3426, 1.934) -> (-37.0239, 1.8314) construction
  line L297 (-37.0239, 1.8314) -> (-36.8076, 1.7667) construction
  line L298 (-36.8076, 1.7667) -> (-36.6984, 1.741) construction
  spline S10 degree 3 poles (-36.6984, 1.741) (-36.6118, 1.7206) (-36.4146, 1.6836) (-36.1334, 1.6511) (-35.8641, 1.6856) (-35.6361, 1.789) (-35.4843, 2.0009) (-35.4107, 2.2607) (-35.4022, 2.5453) (-35.4352, 2.8278) (-35.5538, 3.0859) (-35.7222, 3.2926) (-35.9461, 3.4732) (-36.2017, 3.6197) (-36.4768, 3.7539) (-36.7726, 3.866) (-37.0702, 3.9721) (-37.2825, 4.0233) (-37.3796, 4.0448) knots 0 0 0 0 0.058736 0.132461 0.18557 0.236584 0.29264 0.351158 0.412751 0.479696 0.53687 0.597653 0.654105 0.725762 0.791685 0.855947 0.934442 1 1 1 1
  line L299 (-36.6984, 1.741) -> (-36.6118, 1.7206) construction
  line L300 (-36.6118, 1.7206) -> (-36.4146, 1.6836) construction
  line L301 (-36.4146, 1.6836) -> (-36.1334, 1.6511) construction
  line L302 (-36.1334, 1.6511) -> (-35.8641, 1.6856) construction
  line L303 (-35.8641, 1.6856) -> (-35.6361, 1.789) construction
  line L304 (-35.6361, 1.789) -> (-35.4843, 2.0009) construction
  line L305 (-35.4843, 2.0009) -> (-35.4107, 2.2607) construction
  line L306 (-35.4107, 2.2607) -> (-35.4022, 2.5453) construction
  line L307 (-35.4022, 2.5453) -> (-35.4352, 2.8278) construction
  line L308 (-35.4352, 2.8278) -> (-35.5538, 3.0859) construction
  line L309 (-35.5538, 3.0859) -> (-35.7222, 3.2926) construction
  line L310 (-35.7222, 3.2926) -> (-35.9461, 3.4732) construction
  line L311 (-35.9461, 3.4732) -> (-36.2017, 3.6197) construction
  line L312 (-36.2017, 3.6197) -> (-36.4768, 3.7539) construction
  line L313 (-36.4768, 3.7539) -> (-36.7726, 3.866) construction
  line L314 (-36.7726, 3.866) -> (-37.0702, 3.9721) construction
  line L315 (-37.0702, 3.9721) -> (-37.2825, 4.0233) construction
  line L316 (-37.2825, 4.0233) -> (-37.3796, 4.0448) construction
  spline S11 degree 3 poles (-36.6984, 1.741) (-36.6118, 1.7206) (-36.4146, 1.6836) (-36.1334, 1.6511) (-35.8641, 1.6856) (-35.6361, 1.789) (-35.4843, 2.0009) (-35.4107, 2.2607) (-35.4022, 2.5453) (-35.4352, 2.8278) (-35.5538, 3.0859) (-35.7222, 3.2926) (-35.9461, 3.4732) (-36.2017, 3.6197) (-36.4768, 3.7539) (-36.7726, 3.866) (-37.0702, 3.9721) (-37.2825, 4.0233) (-37.3796, 4.0448) knots 0 0 0 0 0.058736 0.132461 0.18557 0.236584 0.29264 0.351158 0.412751 0.479696 0.53687 0.597653 0.654105 0.725762 0.791685 0.855947 0.934442 1 1 1 1
  line L317 (-36.6984, 1.741) -> (-36.6118, 1.7206) construction
  line L318 (-36.6118, 1.7206) -> (-36.4146, 1.6836) construction
  line L319 (-36.4146, 1.6836) -> (-36.1334, 1.6511) construction
  line L320 (-36.1334, 1.6511) -> (-35.8641, 1.6856) construction
  line L321 (-35.8641, 1.6856) -> (-35.6361, 1.789) construction
  line L322 (-35.6361, 1.789) -> (-35.4843, 2.0009) construction
  line L323 (-35.4843, 2.0009) -> (-35.4107, 2.2607) construction
  line L324 (-35.4107, 2.2607) -> (-35.4022, 2.5453) construction
  line L325 (-35.4022, 2.5453) -> (-35.4352, 2.8278) construction
  line L326 (-35.4352, 2.8278) -> (-35.5538, 3.0859) construction
  line L327 (-35.5538, 3.0859) -> (-35.7222, 3.2926) construction
  line L328 (-35.7222, 3.2926) -> (-35.9461, 3.4732) construction
  line L329 (-35.9461, 3.4732) -> (-36.2017, 3.6197) construction
  line L330 (-36.2017, 3.6197) -> (-36.4768, 3.7539) construction
  line L331 (-36.4768, 3.7539) -> (-36.7726, 3.866) construction
  line L332 (-36.7726, 3.866) -> (-37.0702, 3.9721) construction
  line L333 (-37.0702, 3.9721) -> (-37.2825, 4.0233) construction
  line L334 (-37.2825, 4.0233) -> (-37.3796, 4.0448) construction
  arc A0 (-37.8544, -1.1308) -> (-37.4616, -1.3224) centre (-36.4977, 1.1532) ccw
  arc A1 (-36.7641, -1.5741) -> (-36.2828, -1.7225) centre (-35.1742, 2.7263) ccw
  spline S12 degree 3 poles (-36.7641, -1.5741) (-36.7505, -1.4891) (-36.7247, -1.3264) (-36.7301, -1.0707) (-36.8177, -0.8355) (-37.0007, -0.7186) (-37.1591, -0.6557) (-37.3343, -0.6531) (-37.4608, -0.8025) (-37.4863, -1.0375) (-37.4849, -1.2137) (-37.4616, -1.3224) knots 0.000002 0.000002 0.000002 0.000002 0.130512 0.248338 0.387441 0.486956 0.566128 0.647917 0.731171 0.833817 0.999993 0.999993 0.999993 0.999993
  line L335 (-36.7641, -1.5741) -> (-36.7505, -1.4891) construction
  line L336 (-36.7505, -1.4891) -> (-36.7247, -1.3264) construction
  line L337 (-36.7247, -1.3264) -> (-36.7301, -1.0707) construction
  line L338 (-36.7301, -1.0707) -> (-36.8177, -0.8355) construction
  line L339 (-36.8177, -0.8355) -> (-37.0007, -0.7186) construction
  line L340 (-37.0007, -0.7186) -> (-37.1591, -0.6557) construction
  line L341 (-37.1591, -0.6557) -> (-37.3343, -0.6531) construction
  line L342 (-37.3343, -0.6531) -> (-37.4608, -0.8025) construction
  line L343 (-37.4608, -0.8025) -> (-37.4863, -1.0375) construction
  line L344 (-37.4863, -1.0375) -> (-37.4849, -1.2137) construction
  line L345 (-37.4849, -1.2137) -> (-37.4616, -1.3224) construction
  line L346 (-36.653, 0.7792) -> (-36.5685, 0.7576)
  spline S13 degree 3 poles (-37.8544, -1.1308) (-37.8536, -0.9801) (-37.8499, -0.742) (-37.9125, -0.4332) (-38.0504, -0.2331) (-38.2518, -0.153) (-38.4786, -0.1595) (-38.6195, -0.3387) (-38.6813, -0.5514) (-38.6938, -0.7925) (-38.677, -1.0533) (-38.6261, -1.3179) (-38.5012, -1.5536) (-38.3084, -1.7405) (-38.0832, -1.8914) (-37.839, -2.0089) (-37.5863, -2.1154) (-37.3337, -2.2319) (-37.0666, -2.3111) (-36.8068, -2.3986) (-36.5292, -2.458) (-36.2438, -2.5065) (-35.9696, -2.5082) (-35.7113, -2.4196) (-35.5214, -2.2369) (-35.4217, -1.9412) (-35.3888, -1.645) (-35.4563, -1.3237) (-35.5661, -1.0472) (-35.7908, -0.8405) (-36.0487, -0.7938) (-36.2934, -0.8932) (-36.3899, -1.2666) (-36.3184, -1.5315) (-36.2828, -1.7225) knots 0.000002 0.000002 0.000002 0.000002 0.050812 0.079978 0.105051 0.128715 0.150613 0.176165 0.198359 0.225349 0.256757 0.286428 0.315385 0.345015 0.375912 0.406383 0.43613 0.468337 0.499902 0.529857 0.5606 0.595385 0.627424 0.651669 0.685878 0.711437 0.755573 0.784369 0.821416 0.854265 0.882212 0.905839 0.935385 1 1 1 1
  line L347 (-37.8544, -1.1308) -> (-37.8536, -0.9801) construction
  line L348 (-37.8536, -0.9801) -> (-37.8499, -0.742) construction
  line L349 (-37.8499, -0.742) -> (-37.9125, -0.4332) construction
  line L350 (-37.9125, -0.4332) -> (-38.0504, -0.2331) construction
  line L351 (-38.0504, -0.2331) -> (-38.2518, -0.153) construction
  line L352 (-38.2518, -0.153) -> (-38.4786, -0.1595) construction
  line L353 (-38.4786, -0.1595) -> (-38.6195, -0.3387) construction
  line L354 (-38.6195, -0.3387) -> (-38.6813, -0.5514) construction
  line L355 (-38.6813, -0.5514) -> (-38.6938, -0.7925) construction
  line L356 (-38.6938, -0.7925) -> (-38.677, -1.0533) construction
  line L357 (-38.677, -1.0533) -> (-38.6261, -1.3179) construction
  line L358 (-38.6261, -1.3179) -> (-38.5012, -1.5536) construction
  line L359 (-38.5012, -1.5536) -> (-38.3084, -1.7405) construction
  line L360 (-38.3084, -1.7405) -> (-38.0832, -1.8914) construction
  line L361 (-38.0832, -1.8914) -> (-37.839, -2.0089) construction
  line L362 (-37.839, -2.0089) -> (-37.5863, -2.1154) construction
  line L363 (-37.5863, -2.1154) -> (-37.3337, -2.2319) construction
  line L364 (-37.3337, -2.2319) -> (-37.0666, -2.3111) construction
  line L365 (-37.0666, -2.3111) -> (-36.8068, -2.3986) construction
  line L366 (-36.8068, -2.3986) -> (-36.5292, -2.458) construction
  line L367 (-36.5292, -2.458) -> (-36.2438, -2.5065) construction
  line L368 (-36.2438, -2.5065) -> (-35.9696, -2.5082) construction
  line L369 (-35.9696, -2.5082) -> (-35.7113, -2.4196) construction
  line L370 (-35.7113, -2.4196) -> (-35.5214, -2.2369) construction
  line L371 (-35.5214, -2.2369) -> (-35.4217, -1.9412) construction
  line L372 (-35.4217, -1.9412) -> (-35.3888, -1.645) construction
  line L373 (-35.3888, -1.645) -> (-35.4563, -1.3237) construction
  line L374 (-35.4563, -1.3237) -> (-35.5661, -1.0472) construction
  line L375 (-35.5661, -1.0472) -> (-35.7908, -0.8405) construction
  line L376 (-35.7908, -0.8405) -> (-36.0487, -0.7938) construction
  line L377 (-36.0487, -0.7938) -> (-36.2934, -0.8932) construction
  line L378 (-36.2934, -0.8932) -> (-36.3899, -1.2666) construction
  line L379 (-36.3899, -1.2666) -> (-36.3184, -1.5315) construction
  line L380 (-36.3184, -1.5315) -> (-36.2828, -1.7225) construction
  line L381 (-36.653, 0.7792) -> (-36.5685, 0.7576)
  spline S14 degree 3 poles (-36.295, -3.2208) (-36.3961, -3.1865) (-36.6076, -3.0929) (-36.9302, -2.923) (-37.2988, -2.7694) (-37.6429, -2.612) (-37.947, -2.4624) (-38.2101, -2.395) (-38.4408, -2.3351) (-38.6523, -2.4559) (-38.6702, -2.686) (-38.6453, -2.8298) (-38.6227, -2.8984) knots 0 0 0 0 0.107518 0.23411 0.368721 0.511133 0.617815 0.709418 0.788123 0.85006 0.926906 1 1 1 1
  line L382 (-36.295, -3.2208) -> (-36.3961, -3.1865) construction
  line L383 (-36.3961, -3.1865) -> (-36.6076, -3.0929) construction
  line L384 (-36.6076, -3.0929) -> (-36.9302, -2.923) construction
  line L385 (-36.9302, -2.923) -> (-37.2988, -2.7694) construction
  line L386 (-37.2988, -2.7694) -> (-37.6429, -2.612) construction
  line L387 (-37.6429, -2.612) -> (-37.947, -2.4624) construction
  line L388 (-37.947, -2.4624) -> (-38.2101, -2.395) construction
  line L389 (-38.2101, -2.395) -> (-38.4408, -2.3351) construction
  line L390 (-38.4408, -2.3351) -> (-38.6523, -2.4559) construction
  line L391 (-38.6523, -2.4559) -> (-38.6702, -2.686) construction
  line L392 (-38.6702, -2.686) -> (-38.6453, -2.8298) construction
  line L393 (-38.6453, -2.8298) -> (-38.6227, -2.8984) construction
  spline S15 degree 3 poles (-38.6227, -2.8984) (-38.5671, -3.0675) (-38.3501, -3.2221) (-38.0283, -3.3874) (-37.7632, -3.5103) (-37.4823, -3.6447) (-37.1771, -3.7647) (-36.8447, -3.8847) (-36.5182, -4.002) (-36.1996, -4.0704) (-35.8996, -4.1189) (-35.6034, -4.042) (-35.4212, -3.7695) (-35.4175, -3.442) (-35.4429, -3.1128) (-35.5754, -2.8248) (-35.7947, -2.6631) (-36.0051, -2.6098) (-36.201, -2.6189) (-36.2695, -2.7587) (-36.3466, -2.9422) (-36.295, -3.1086) (-36.295, -3.2208) knots 0 0 0 0 0.084367 0.132854 0.185682 0.233817 0.292249 0.353411 0.414803 0.469553 0.519939 0.570079 0.615873 0.676082 0.733974 0.784619 0.833154 0.866506 0.897762 0.921095 0.940031 1 1 1 1
  line L394 (-38.6227, -2.8984) -> (-38.5671, -3.0675) construction
  line L395 (-38.5671, -3.0675) -> (-38.3501, -3.2221) construction
  line L396 (-38.3501, -3.2221) -> (-38.0283, -3.3874) construction
  line L397 (-38.0283, -3.3874) -> (-37.7632, -3.5103) construction
  line L398 (-37.7632, -3.5103) -> (-37.4823, -3.6447) construction
  line L399 (-37.4823, -3.6447) -> (-37.1771, -3.7647) construction
  line L400 (-37.1771, -3.7647) -> (-36.8447, -3.8847) construction
  line L401 (-36.8447, -3.8847) -> (-36.5182, -4.002) construction
  line L402 (-36.5182, -4.002) -> (-36.1996, -4.0704) construction
  line L403 (-36.1996, -4.0704) -> (-35.8996, -4.1189) construction
  line L404 (-35.8996, -4.1189) -> (-35.6034, -4.042) construction
  line L405 (-35.6034, -4.042) -> (-35.4212, -3.7695) construction
  line L406 (-35.4212, -3.7695) -> (-35.4175, -3.442) construction
  line L407 (-35.4175, -3.442) -> (-35.4429, -3.1128) construction
  line L408 (-35.4429, -3.1128) -> (-35.5754, -2.8248) construction
  line L409 (-35.5754, -2.8248) -> (-35.7947, -2.6631) construction
  line L410 (-35.7947, -2.6631) -> (-36.0051, -2.6098) construction
  line L411 (-36.0051, -2.6098) -> (-36.201, -2.6189) construction
  line L412 (-36.201, -2.6189) -> (-36.2695, -2.7587) construction
  line L413 (-36.2695, -2.7587) -> (-36.3466, -2.9422) construction
  line L414 (-36.3466, -2.9422) -> (-36.295, -3.1086) construction
  line L415 (-36.295, -3.1086) -> (-36.295, -3.2208) construction
  spline S16 degree 3 poles (-36.4459, 2.4614) (-36.659, 2.5126) (-37.0118, 2.6203) (-37.4792, 2.8097) (-37.7435, 2.9186) (-37.8615, 2.9876) knots 0 0 0 0 0.434487 0.729459 1 1 1 1
  line L416 (-36.4459, 2.4614) -> (-36.659, 2.5126) construction
  line L417 (-36.659, 2.5126) -> (-37.0118, 2.6203) construction
  line L418 (-37.0118, 2.6203) -> (-37.4792, 2.8097) construction
  line L419 (-37.4792, 2.8097) -> (-37.7435, 2.9186) construction
  line L420 (-37.7435, 2.9186) -> (-37.8615, 2.9876) construction
  spline S17 degree 3 poles (-37.8615, 2.9876) (-37.8896, 3.004) (-37.9483, 3.0417) (-38.008, 3.1224) (-38.013, 3.2088) (-38.0172, 3.2823) (-37.9686, 3.355) (-37.867, 3.3615) (-37.7329, 3.3463) (-37.555, 3.298) (-37.3426, 3.2417) (-37.1448, 3.173) (-36.9458, 3.1066) (-36.7442, 3.0312) (-36.534, 2.9393) (-36.3445, 2.8534) (-36.1878, 2.7622) (-36.1364, 2.6314) (-36.1459, 2.5251) (-36.2475, 2.422) (-36.3751, 2.4459) (-36.4459, 2.4614) knots 0 0 0 0 0.033985 0.073024 0.098291 0.123366 0.14909 0.179483 0.222309 0.292562 0.370552 0.452514 0.511152 0.58996 0.677574 0.750224 0.809779 0.859921 0.887962 0.916689 1 1 1 1
  line L421 (-37.8615, 2.9876) -> (-37.8896, 3.004) construction
  line L422 (-37.8896, 3.004) -> (-37.9483, 3.0417) construction
  line L423 (-37.9483, 3.0417) -> (-38.008, 3.1224) construction
  line L424 (-38.008, 3.1224) -> (-38.013, 3.2088) construction
  line L425 (-38.013, 3.2088) -> (-38.0172, 3.2823) construction
  line L426 (-38.0172, 3.2823) -> (-37.9686, 3.355) construction
  line L427 (-37.9686, 3.355) -> (-37.867, 3.3615) construction
  line L428 (-37.867, 3.3615) -> (-37.7329, 3.3463) construction
  line L429 (-37.7329, 3.3463) -> (-37.555, 3.298) construction
  line L430 (-37.555, 3.298) -> (-37.3426, 3.2417) construction
  line L431 (-37.3426, 3.2417) -> (-37.1448, 3.173) construction
  line L432 (-37.1448, 3.173) -> (-36.9458, 3.1066) construction
  line L433 (-36.9458, 3.1066) -> (-36.7442, 3.0312) construction
  line L434 (-36.7442, 3.0312) -> (-36.534, 2.9393) construction
  line L435 (-36.534, 2.9393) -> (-36.3445, 2.8534) construction
  line L436 (-36.3445, 2.8534) -> (-36.1878, 2.7622) construction
  line L437 (-36.1878, 2.7622) -> (-36.1364, 2.6314) construction